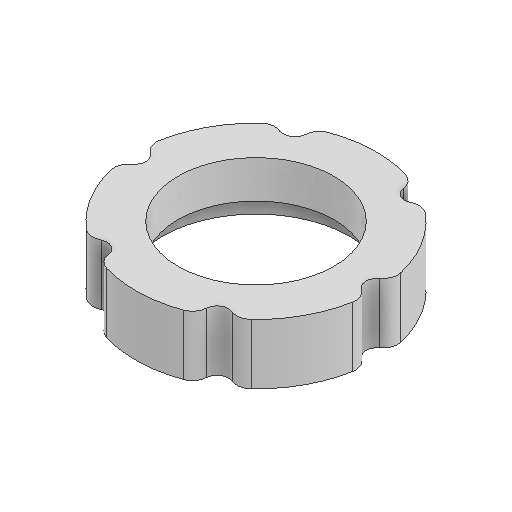
# Autodesk Inventor part: springSpacerV1
Saved by Autodesk Inventor 2025 (Build 290162000, 162)
## iProperties
Created: 2024-11-07
Part Number: springSpacerV1
Material: Generic
Document SubType Name: Modeling
Designer: derm
Density: 1 g/cm^3
Appearance: Default
Author: derm
Autodesk Inventor part; units mm, degrees
ref_plane "YZ Plane" through (0, 0, 0) normal (1, 0, 0) x (0, 1, 0)
ref_plane "XZ Plane" through (0, 0, 0) normal (0, 1, 0) x (-1, 0, 0)
ref_plane "XY Plane" through (0, 0, 0) normal (0, 0, 1) x (1, 0, 0)
sketch "Sketch1" plane through (0, 0, 0) normal (0, 1, 0) x (-1, 0, 0)
  circle A0 centre (0, 0) radius 10.375
  arc A1 (15.885, 1.9145) -> (15.9655, -1.0494) centre (15.6971, 0.4263) ccw
  arc A2 (6.2845, 14.7141) -> (8.8916, 13.3018) centre (7.4793, 13.8073) ccw
  arc A3 (-9.6005, 12.7996) -> (-7.0739, 14.3513) centre (-8.2178, 13.3809) ccw
  arc A4 (-15.885, -1.9145) -> (-15.9655, 1.0494) centre (-15.6971, -0.4263) ccw
  arc A5 (-6.2845, -14.7141) -> (-8.8916, -13.3018) centre (-7.4793, -13.8073) ccw
  arc A6 (9.6005, -12.7996) -> (7.0739, -14.3513) centre (8.2178, -13.3809) ccw
  arc A7 (9.6005, -12.7996) -> (15.9655, -1.0494) centre (0, 0) ccw
  arc A8 (-6.2845, -14.7141) -> (7.0739, -14.3513) centre (0, 0) ccw
  arc A9 (-15.885, -1.9145) -> (-8.8916, -13.3018) centre (0, 0) ccw
  arc A10 (-9.6005, 12.7996) -> (-15.9655, 1.0494) centre (0, 0) ccw
  arc A11 (15.885, 1.9145) -> (8.8916, 13.3018) centre (0, 0) ccw
  arc A12 (6.2845, 14.7141) -> (-7.0739, 14.3513) centre (0, 0) ccw
  dimension "d0" = 20.75
  dimension "d4" = 3
  dimension "d7" = 360
  dimension "d10" = 16
  constraints: 24 point on circle, 13 centre point, 2 coincident, 25 other
  measures "d0" diameter of A0
  measures "d4" diameter of A1
  measures "d10" radius of A11
extrude "Extrusion1" add sketch "Sketch1" along normal blind 8
fillet "Fillet1" radius 2 12 edges at (9.6005, 4, 12.7996) (15.9655, 4, 1.0494) (15.885, 4, -1.9145) (8.8916, 4, -13.3018) (6.2845, 4, -14.7141) (-7.0739, 4, -14.3513) (-9.6005, 4, -12.7996) (-15.9655, 4, -1.0494) (-15.885, 4, 1.9145) (-8.8916, 4, 13.3018) (-6.2845, 4, 14.7141) (7.0739, 4, 14.3513)
sketch "Sketch2" plane through (0, 0, 0) normal (0, -1, 0) x (1, 0, 0)
  circle A0 centre (0, 0) radius 10.375 projected
  circle A1 centre (0, 0) radius 12.5
  dimension "d11" = 25
  constraints: 1 centre point, 1 coincident
  measures "d11" diameter of A1
extrude "Extrusion2" cut sketch "Sketch2" against normal blind 3
body "Solid1"
